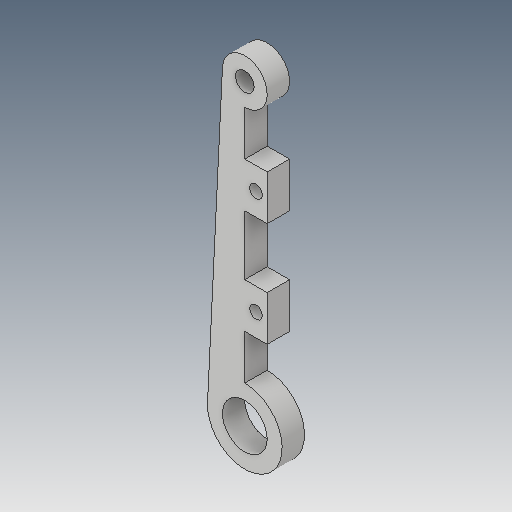
# Autodesk Inventor part: link1
Saved by Autodesk Inventor 2019.4 (Build 234330000, 330)
## iProperties
Created: 2018-08-30
Part Number: link1
Material: 一般
Document SubType Name: Modeling
Designer: AzLIer
Density: 1 g/cm^3
Appearance: 既定
Author: AzLIer
Autodesk Inventor part; units mm, degrees
ref_plane "YZ Plane" through (0, 0, 0) normal (1, 0, 0) x (0, 1, 0)
ref_plane "XZ Plane" through (0, 0, 0) normal (0, 1, 0) x (-1, 0, 0)
ref_plane "XY Plane" through (0, 0, 0) normal (0, 0, 1) x (1, 0, 0)
sketch "スケッチ1" plane through (0, 0, 0) normal (0, 0, 1) x (1, 0, 0)
  circle A0 centre (0, 0) radius 3
  circle A1 centre (0, 40) radius 1.25
  circle A2 centre (0, 40) radius 3
  circle A3 centre (0, 0) radius 5
  line L0 (0, 5) -> (0, 37)
  line L1 (-2.9962, 40.15) -> (-4.9937, 0.25)
  dimension "d0" = 6
  dimension "d1" = 2.5
  dimension "d2" = 40
  dimension "d3" = 6
  dimension "d4" = 10
  constraints: 4 centre point, 4 end point, 4 point on circle, 2 coincident, 2 tangent, 1 point on line, 1 vertical, 1 vertical alignment
  measures "d0" diameter of A0
  measures "d1" diameter of A1
  measures "d2" distance of point (0, 0) A1.centre
  measures "d3" diameter of A2
  measures "d4" diameter of A3
extrude "押し出し1" add sketch "スケッチ1" along normal blind 3
sketch "スケッチ2" plane through (0, 0, 3) normal (0, 0, 1) x (1, 0, 0)
  circle A0 centre (0, 0) radius 3 projected
  circle A1 centre (0, 40) radius 1.25 projected
  arc A2 (0, 37) -> (-2.9962, 40.15) centre (0, 40) ccw projected
  line L0 (-2.9962, 40.15) -> (-4.9937, 0.25) projected
  arc A3 (-4.9937, 0.25) -> (0, 5) centre (0, 0) ccw projected
  line L1 (0, 5) -> (0, 37) projected
  circle A4 centre (0, 0) radius 3
  circle A5 centre (-32.1289, 23.8272) radius 1.25
  line L2 (-4.0161, 2.9784) -> (-4.827, 3.5798)
  arc A6 (-30.4645, 26.3232) -> (-29.7192, 22.0402) centre (-32.1289, 23.8272) ccw
  line L3 (-4.5534, 9.0458) -> (2.7739, 4.16)
  arc A7 (-4.0161, 2.9784) -> (2.7739, 4.16) centre (0, 0) ccw
  constraints: 4 centre point, 4 end point, 4 point on circle, 2 point on line, 14 other
extrude "押し出し2" [suppressed]
sketch "スケッチ4" plane through (0, 0, 3) normal (0, 0, 1) x (1, 0, 0)
  line L0 (-4.9937, 0.25) -> (-2.9962, 40.15) projected
  arc A0 (0, 37) -> (-2.9962, 40.15) centre (0, 40) ccw projected
  line L1 (0, 37) -> (0, 5) projected
  circle A1 centre (0, 40) radius 1.25 projected
  circle A2 centre (-27.9404, 11.376) radius 3
  circle A3 centre (0, 40) radius 1.25
  line L2 (-3.1661, 36.7564) -> (-2.0955, 37.8532)
  arc A4 (2.2489, 38.0144) -> (-2.0955, 37.8532) centre (0, 40) ccw
  line L3 (2.2489, 38.0144) -> (-3.4249, 31.5882)
  arc A5 (-24.4479, 14.954) -> (-24.1923, 8.0667) centre (-27.9404, 11.376) ccw
  circle A6 centre (0, 0) radius 3 projected
  arc A7 (-4.9937, 0.25) -> (0, 5) centre (0, 0) ccw projected
  constraints: 4 centre point, 4 end point, 4 point on circle, 2 point on line, 14 other
extrude "押し出し3" [suppressed]
sketch "スケッチ5" plane through (0, 0, 3) normal (0, 0, 1) x (1, 0, 0)
  circle A0 centre (0, 0) radius 3 projected
  circle A1 centre (0, 40) radius 1.25 projected
  arc A2 (0, 37) -> (-2.9962, 40.15) centre (0, 40) ccw projected
  line L0 (-2.9962, 40.15) -> (-4.9937, 0.25) projected
  arc A3 (-4.9937, 0.25) -> (0, 5) centre (0, 0) ccw projected
  line L1 (0, 5) -> (0, 37) projected
  line L2 (0, 31) -> (3, 31)
  line L3 (3, 31) -> (3, 25)
  line L4 (3, 25) -> (0, 25)
  line L5 (0, 17) -> (3, 17)
  line L6 (3, 17) -> (3, 11)
  line L7 (3, 11) -> (0, 11)
  circle A4 centre (1.5, 14) radius 0.85
  circle A5 centre (1.5, 28) radius 0.85
  point P0 (1.5, 31)
  point P1 (1.5, 17)
  point P2 (3, 28)
  point P3 (3, 14)
  dimension "d12" = 6
  dimension "d13" = 3
  dimension "d14" = 8
  dimension "d15" = 6
  dimension "d16" = 6
  dimension "d19" = 1.7
  constraints: 12 end point, 5 perpendicular, 4 midpoint, 4 point on line, 2 centre point, 2 equal length, 2 horizontal alignment, 2 vertical alignment, 1 equal radius, 1 horizontal
  measures "d12" distance of L2.end L3.end
  measures "d13" distance of L2.start L2.end
  measures "d14" distance between parallel lines of L5 L4
  measures "d15" distance from line of L2 L1.end
  measures "d16" distance from line of L1.start L7
  measures "d19" diameter of A5
extrude "押し出し4" add sketch "スケッチ5" against normal blind 3 contours L2 L3 L4 L1 | L5 L6 L7 L1
equation "\"d15\" = d16"
